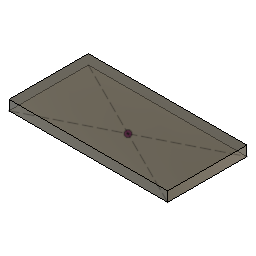
Assembly (Autodesk Fusion 360 archive; units mm, degrees)
design "PDMS Chip"
Autodesk Fusion 360 part; units mm, degrees
sketch "Sketch1" plane through (0, 0, 0) normal (0, 0, 1) x (1, 0, 0)
  line L0 (20, -10) -> (-20, -10)
  line L1 (-20, -10) -> (-20, 10)
  line L2 (-20, 10) -> (20, 10)
  line L3 (20, 10) -> (20, -10)
  line L4 (20, -10) -> (-20, 10) construction
  line L5 (-20, -10) -> (20, 10) construction
  dimension "d1" = 40
  dimension "d2" = 20
  constraint perpendicular L0 L1
  constraint parallel L0 L2
  constraint parallel L1 L3
  constraint horizontal L0
  constraint coincident L4 origin
  constraint coincident L5 origin
  measures "d1" distance of L1.end L2.end
  measures "d2" distance of L0.start L2.end
extrude "Extrude1" add sketch "Sketch1" along normal blind 2.5

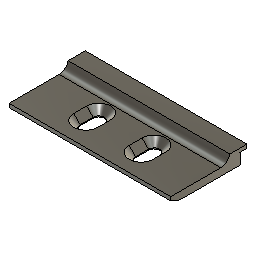
design "Microfluidic Clamp"
Autodesk Fusion 360 part; units mm, degrees
sketch "Sketch1" plane through (0, 0, 0) normal (0, 0, 1) x (1, 0, 0)
  line L0 (17.5, -7.5) -> (-17.5, -7.5)
  line L1 (-17.5, -7.5) -> (-17.5, 7.5)
  line L2 (-17.5, 7.5) -> (17.5, 7.5)
  line L3 (17.5, 7.5) -> (17.5, -7.5)
  line L4 (17.5, -7.5) -> (-17.5, 7.5) construction
  line L5 (-17.5, -7.5) -> (17.5, 7.5) construction
  dimension "d1" = 35
  dimension "d2" = 15
  constraint perpendicular L0 L1
  constraint parallel L0 L2
  constraint parallel L1 L3
  constraint horizontal L0
  constraint coincident L4 origin
  constraint coincident L5 origin
  measures "d1" distance of L1.end L2.end
  measures "d2" distance of L0.start L2.end
extrude "Extrude1" add sketch "Sketch1" along normal blind 1.6
sketch "Sketch2" plane through (17.5, 0, 0) normal (1, 0, 0) x (0, 1, 0)
  line L0 (-7.5, 0) -> (7.5, 0)
  line L1 (7.5, 0) -> (7.5, 1.6)
  line L2 (7.5, 1.6) -> (-7.5, 1.6)
  line L3 (-7.5, 1.6) -> (-7.5, 0)
  line L4 (-5.5, 0) -> (-7.5, 0.8)
  line L5 (-7.5, 0.8) -> (-7.5, 0)
  line L6 (-7.5, 0) -> (-5.5, 0)
  dimension "d5" = 2
  constraint coincident L0 L4.start
  constraint midpoint L3 L4.end
  constraint coincident L0.start L3.end
  measures "d5" distance of L4.start L0.start
extrude "Extrude2" cut sketch "Sketch2" against normal up to surface (35 mm away) contours L0 L3 L4 L5 L6
sketch "Sketch3" plane through (0, 0, 1.6) normal (0, 0, 1) x (-1, 0, 0)
  line L0 (-17.5, -7.5) -> (17.5, -7.5)
  line L1 (17.5, -7.5) -> (17.5, 7.5)
  line L2 (17.5, 7.5) -> (-17.5, 7.5)
  line L3 (-17.5, 7.5) -> (-17.5, -7.5)
  line L4 (17.5, -7.5) -> (-17.5, -7.5)
  line L5 (-17.5, -7.5) -> (-17.5, -5.3)
  line L6 (-17.5, -5.3) -> (17.5, -5.3)
  line L7 (17.5, -5.3) -> (17.5, -7.5)
  dimension "d8" = 2.2
  constraint horizontal L4
  constraint vertical L5
  constraint horizontal L6
  constraint vertical L7
  constraint coincident L3 L5.end
  constraint coincident L0.end L1.start
  measures "d8" distance of L0.start L5.end
extrude "Extrude3" add sketch "Sketch3" along normal blind 1.6 contours L0 L1 L3 L4 L5 L6 L7
fillet "Fillet1" radius 2 1 edges at (0, 5.3, 1.6)
sketch "Sketch4" plane through (0, 7.5, 0) normal (0, 1, 0) x (-1, 0, 0)
  line L0 (-17.5, 0) -> (17.5, 0)
  line L1 (17.5, 0) -> (17.5, 3.2)
  line L2 (17.5, 3.2) -> (-17.5, 3.2)
  line L3 (-17.5, 3.2) -> (-17.5, 0)
  line L4 (-17.5, 3.2) -> (17.5, 3.2)
  line L5 (17.5, 3.2) -> (17.5, 2.4)
  line L6 (17.5, 2.4) -> (-17.5, 2.4)
  line L7 (-17.5, 2.4) -> (-17.5, 3.2)
  line L8 (17.5, 1.6) -> (17.5, 3.2)
  dimension "d12" = 1
  constraint horizontal L4
  constraint vertical L5
  constraint horizontal L6
  constraint vertical L7
  constraint midpoint L5.end L8
  constraint coincident L2.end L3.start
extrude "Extrude4" add sketch "Sketch4" along normal blind 1.5 contours L1 L2 L3 L4 L5 L6 L7 L8
sketch "Sketch5" plane through (0, 0, 1.6) normal (0, 0, 1) x (-1, 0, 0)
  line L0 (-17.5, -3.3404) -> (17.5, -3.3404)
  line L1 (17.5, -3.3404) -> (17.5, 7.5)
  line L2 (17.5, 7.5) -> (-17.5, 7.5)
  line L3 (-17.5, 7.5) -> (-17.5, -3.3404)
  line L4 (6, 1) -> (-6, 1)
  line L5 (4.8, 2.4) -> (7.2, 2.4)
  line L6 (7.2, 2.4) -> (7.2, -0.4)
  line L7 (7.2, -0.4) -> (4.8, -0.4)
  line L8 (4.8, -0.4) -> (4.8, 2.4)
  line L9 (4.8, 2.4) -> (7.2, -0.4) construction
  line L10 (7.2, 2.4) -> (4.8, -0.4) construction
  arc A0 (4.8, -0.4) -> (7.2, -0.4) centre (6, -0.4) ccw
  arc A1 (7.2, 2.4) -> (4.8, 2.4) centre (6, 2.4) ccw
  line L11 (0, -1.5) -> (0, 7.5)
  arc A2 (-4.8, 2.4) -> (-7.2, 2.4) centre (-6, 2.4) ccw
  arc A3 (-7.2, -0.4) -> (-4.8, -0.4) centre (-6, -0.4) ccw
  line L12 (-4.8, 2.4) -> (-7.2, 2.4)
  line L13 (-4.8, 2.4) -> (-7.2, -0.4) construction
  line L14 (-4.8, -0.4) -> (-4.8, 2.4)
  line L15 (-7.2, 2.4) -> (-7.2, -0.4)
  line L16 (-7.2, 2.4) -> (-4.8, -0.4) construction
  line L17 (-7.2, -0.4) -> (-4.8, -0.4)
  line L18 (17.5, -7.5) -> (-17.5, -7.5)
  point P0 (0, 1)
  point P1 (6, 1)
  point P2 (-6, 1)
  point P3 (-6, 1)
  dimension "d15" = 12
  dimension "d18" = 2.4
  dimension "d19" = 2.8
  dimension "d20" = 1.2
  dimension "d21" = 1.2
  dimension "d25" = 8.5
  constraint parallel L0 L4
  constraint midpoint L4 P0
  constraint vertical origin P0
  constraint perpendicular L5 L6
  constraint parallel L5 L7
  constraint parallel L6 L8
  constraint horizontal L5
  constraint coincident L9 P1
  constraint coincident L10 P1
  constraint coincident P1 L4.start
  constraint midpoint L7 A0.centre
  constraint midpoint L5 A1.centre
  constraint midpoint L2 L11.end
  constraint perpendicular L2 L11
  constraint symmetric P1 L11 P3
  constraint symmetric L5.start L11 A2.start
  constraint symmetric L5.end L11 A2.end
  constraint symmetric L6.end L11 A3.start
  constraint symmetric L7.end L11 A3.end
  constraint symmetric A0 L11 A3
  constraint symmetric A1 L11 A2
  measures "d15" distance of P1 P3
  measures "d18" distance of L5.start L5.end
  measures "d19" distance of L5.end L6.end
  measures "d20" radius of A0
  measures "d21" radius of A1
  measures "d25" distance of L4 L18
extrude "Extrude5" cut sketch "Sketch5" against normal up to surface (1.6 mm away) contours L5 A1 | L5 L6 L7 L8 | L7 A0 | A2 L12 | L12 L14 L15 L17 | A3 L17
chamfer "Chamfer1" distance 1.4 angle 45 8 edges at (-6, -3.6, 1.6) (-7.2, -1, 1.6) (-6, 1.6, 1.6) (-4.8, -1, 1.6) (4.8, -1, 1.6) (6, 1.6, 1.6) (7.2, -1, 1.6) (6, -3.6, 1.6)
fillet "Fillet2" radius 1 1 edges at (0, -5.5, 0)

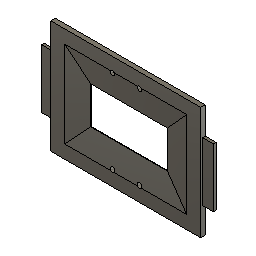
design "Microfluidic TIRF Support"
Autodesk Fusion 360 part; units mm, degrees
sketch "Sketch1" plane through (0, 0, 0) normal (0, 0, 1) x (1, 0, 0) in component "TIRF Support"
  line L0 (0, 0) -> (76, 0)
  line L1 (76, 0) -> (76, 50)
  line L2 (76, 50) -> (0, 50)
  line L3 (0, 50) -> (0, 0)
  line L4 (4.8, 38) -> (-4.8, 38)
  line L5 (-4.8, 38) -> (-4.8, 12)
  line L6 (-4.8, 12) -> (4.8, 12)
  line L7 (4.8, 12) -> (4.8, 38)
  line L8 (4.8, 38) -> (-4.8, 12) construction
  line L9 (-4.8, 38) -> (4.8, 12) construction
  line L10 (71.2, 38) -> (80.8, 38)
  line L11 (80.8, 38) -> (80.8, 12)
  line L12 (80.8, 12) -> (71.2, 12)
  line L13 (71.2, 12) -> (71.2, 38)
  line L14 (71.2, 38) -> (80.8, 12) construction
  line L15 (80.8, 38) -> (71.2, 12) construction
  line L16 (4.8, 50) -> (4.8, 0)
  line L17 (71.2, 50) -> (71.2, 0)
  line L18 (4.8, 0) -> (71.2, 50) construction
  line L19 (4.8, 50) -> (71.2, 0) construction
  point P0 (0, 25)
  point P1 (76, 25)
  point P2 (38, 25)
  dimension "d1" = 76
  dimension "d2" = 50
  dimension "d3" = 26
  dimension "d4" = 26
  dimension "d5" = 4.8
  dimension "d6" = 4.8
  constraint horizontal L0
  constraint vertical L1
  constraint horizontal L2
  constraint vertical L3
  constraint coincident L0.start L3.end
  constraint perpendicular L4 L5
  constraint parallel L4 L6
  constraint parallel L5 L7
  constraint horizontal L4
  constraint coincident L8 P0
  constraint coincident L9 P0
  constraint midpoint L3 P0
  constraint perpendicular L10 L11
  constraint parallel L10 L12
  constraint parallel L11 L13
  constraint horizontal L10
  constraint coincident L14 P1
  constraint coincident L15 P1
  constraint midpoint L1 P1
  constraint coincident L2 L16.start
  constraint coincident L0 L16.end
  constraint perpendicular L0 L16
  constraint coincident L2 L17.start
  constraint perpendicular L2 L17
  constraint coincident L0 L17.end
  constraint collinear L7 L16
  constraint collinear L13 L17
  constraint midpoint L18 P2
  measures "d1" horizontal distance of L0.start L0.end
  measures "d2" vertical distance of L0.start L2.end
  measures "d3" vertical distance of L4.end L5.end
  measures "d4" vertical distance of L10.end L11.end
  measures "d5" distance of L3 L6.end
  measures "d6" distance of L1 L11
extrude "Extrude1" add sketch "Sketch1" along normal blind 2 contours L0 L2 L7 L13 L16 L17 | L3 L4 L6 L7 L16 | L1 L10 L12 L13 L17 in component "TIRF Support"
sketch "Sketch2" plane through (0, 0, 2) normal (0, 0, 1) x (1, 0, 0) in component "TIRF Support"
  line L0 (4.8, 50) -> (4.8, 38)
  line L1 (4.8, 38) -> (0, 38)
  line L2 (0, 38) -> (0, 12)
  line L3 (0, 12) -> (4.8, 12)
  line L4 (4.8, 12) -> (4.8, 0)
  line L5 (4.8, 0) -> (71.2, 0)
  line L6 (71.2, 0) -> (71.2, 12)
  line L7 (71.2, 12) -> (76, 12)
  line L8 (76, 12) -> (76, 38)
  line L9 (76, 38) -> (71.2, 38)
  line L10 (71.2, 38) -> (71.2, 50)
  line L11 (71.2, 50) -> (4.8, 50)
  line L12 (0, 38) -> (4.8, 38)
  line L13 (4.8, 38) -> (4.8, 12)
  line L14 (4.8, 12) -> (0, 12)
  line L15 (0, 12) -> (0, 38)
  line L16 (71.2, 12) -> (76, 12)
  line L17 (76, 12) -> (76, 38)
  line L18 (76, 38) -> (71.2, 38)
  line L19 (71.2, 38) -> (71.2, 12)
  constraint horizontal L12
  constraint vertical L13
  constraint horizontal L14
  constraint vertical L15
  constraint coincident L3.end L4.start
  constraint coincident L1.end L2.start
  constraint horizontal L16
  constraint vertical L17
  constraint horizontal L18
  constraint vertical L19
  constraint coincident L8.end L9.start
  constraint coincident L6.end L7.start
extrude "Extrude2" cut sketch "Sketch2" against normal blind 0.8 contours L1 L2 L3 L12 L13 L14 L15 | L7 L8 L9 L16 L17 L18 L19 in component "TIRF Support"
sketch "Sketch3" plane through (0, 0, 0) normal (0, 0, 1) x (1, 0, 0) in component "TIRF Support"
  line L0 (71.2, 0) -> (4.8, 50)
  line L1 (4.8, 0) -> (71.2, 50)
  line L2 (17.75, 13.75) -> (58.25, 13.75)
  line L3 (58.25, 13.75) -> (58.25, 36.25)
  line L4 (58.25, 36.25) -> (17.75, 36.25)
  line L5 (17.75, 36.25) -> (17.75, 13.75)
  line L6 (17.75, 13.75) -> (58.25, 36.25) construction
  line L7 (58.25, 13.75) -> (17.75, 36.25) construction
  point P0 (71.2, 0)
  point P1 (4.8, 50)
  point P2 (4.8, 0)
  point P3 (71.2, 50)
  point P4 (38, 25)
  dimension "d11" = 22.5
  dimension "d12" = 40.5
  constraint coincident P0 L0.start
  constraint coincident P1 L0.end
  constraint coincident P2 L1.start
  constraint coincident P3 L1.end
  constraint perpendicular L2 L3
  constraint parallel L2 L4
  constraint parallel L3 L5
  constraint horizontal L2
  constraint coincident L6 P4
  constraint coincident L7 P4
  constraint midpoint L1 P4
  measures "d11" vertical distance of L2.end L3.end
  measures "d12" horizontal distance of L2.start L2.end
extrude "Extrude3" cut sketch "Sketch3" along normal blind 0.3 in component "TIRF Support"
sketch "Sketch4" plane through (0, 0, 0.3) normal (0, 0, -1) x (-1, 0, 0) in component "TIRF Support"
  line L0 (-17.75, 13.75) -> (-17.75, 36.25)
  line L1 (-17.75, 36.25) -> (-58.25, 36.25)
  line L2 (-58.25, 36.25) -> (-58.25, 13.75)
  line L3 (-58.25, 13.75) -> (-17.75, 13.75)
  line L4 (-58.25, 13.75) -> (-17.75, 36.25) construction
  line L5 (-58.25, 36.25) -> (-17.75, 13.75) construction
  line L6 (-21, 16.75) -> (-55, 16.75)
  line L7 (-55, 16.75) -> (-55, 33.25)
  line L8 (-55, 33.25) -> (-21, 33.25)
  line L9 (-21, 33.25) -> (-21, 16.75)
  line L10 (-21, 16.75) -> (-55, 33.25) construction
  line L11 (-55, 16.75) -> (-21, 33.25) construction
  point P0 (-38, 25)
  dimension "d15" = 34
  dimension "d16" = 16.5
  constraint coincident L2.end L3.start
  constraint coincident L0.end L1.start
  constraint coincident L1.end L2.start
  constraint coincident L0.start L3.end
  constraint perpendicular L6 L7
  constraint parallel L6 L8
  constraint parallel L7 L9
  constraint horizontal L6
  constraint coincident L10 P0
  constraint coincident L11 P0
  constraint midpoint L4 P0
  measures "d15" horizontal distance of L6.start L6.end
  measures "d16" vertical distance of L6.end L7.end
extrude "Extrude7" cut sketch "Sketch4" against normal blind 0.25 contours L6 L7 L8 L9 in component "TIRF Support"
sketch "Sketch5" plane through (0, 0, 2) normal (0, 0, 1) x (1, 0, 0) in component "TIRF Support"
  line L0 (4.8, 50) -> (4.8, 0)
  line L1 (4.8, 0) -> (71.2, 0)
  line L2 (71.2, 0) -> (71.2, 50)
  line L3 (71.2, 50) -> (4.8, 50)
  line L4 (65, 44.141) -> (11, 44.141)
  line L5 (11, 44.141) -> (11, 5.859)
  line L6 (11, 5.859) -> (65, 5.859)
  line L7 (65, 5.859) -> (65, 44.141)
  line L8 (65, 44.141) -> (11, 5.859) construction
  line L9 (11, 44.141) -> (65, 5.859) construction
  line L10 (21, 33.25) -> (21, 16.75)
  point P0 (38, 25)
  point P1 (38, 25)
  dimension "d18" = 38.282
  dimension "d74" = 10
  constraint perpendicular L4 L5
  constraint parallel L4 L6
  constraint parallel L5 L7
  constraint horizontal L4
  constraint coincident L8 P1
  constraint coincident L9 P1
  constraint coincident P1 P0
  measures "d18" vertical distance of L4.end L5.end
  measures "d74" distance of L5 L10
sketch "Sketch2 (2)" plane through (0, 0, 0) normal (0, 0, -1) x (-1, 0, 0)
  line L0 (-58.25, 36.25) -> (-17.75, 36.25)
  line L1 (-17.75, 36.25) -> (-17.75, 13.75)
  line L2 (-17.75, 13.75) -> (-58.25, 13.75)
  line L3 (-58.25, 13.75) -> (-58.25, 36.25)
  line L4 (-4.8, 38) -> (-4.8, 50)
  line L5 (-4.8, 50) -> (-71.2, 50)
  line L6 (-71.2, 50) -> (-71.2, 38)
  line L7 (-71.2, 38) -> (-76, 38)
  line L8 (-76, 38) -> (-76, 12)
  line L9 (-76, 12) -> (-71.2, 12)
  line L10 (-71.2, 12) -> (-71.2, 0)
  line L11 (-71.2, 0) -> (-4.8, 0)
  line L12 (-4.8, 0) -> (-4.8, 12)
  line L13 (-4.8, 12) -> (0, 12)
  line L14 (0, 12) -> (0, 38)
  line L15 (0, 38) -> (-4.8, 38)
  line L16 (-58.25, 40.25) -> (-54.25, 40.25)
  line L17 (-54.25, 40.25) -> (-54.25, 9.75)
  line L18 (-54.25, 9.75) -> (-58.25, 9.75)
  line L19 (-58.25, 9.75) -> (-58.25, 40.25)
  line L20 (-17.75, 40.25) -> (-21.75, 40.25)
  line L21 (-21.75, 40.25) -> (-21.75, 9.75)
  line L22 (-21.75, 9.75) -> (-17.75, 9.75)
  line L23 (-17.75, 9.75) -> (-17.75, 40.25)
  dimension "d38" = 4
  dimension "d39" = 4
  dimension "d40" = 4
  dimension "d41" = 4
  dimension "d42" = 4
  dimension "d43" = 4
  constraint perpendicular L16 L17
  constraint parallel L16 L18
  constraint parallel L17 L19
  constraint perpendicular L20 L21
  constraint parallel L20 L22
  constraint parallel L21 L23
  constraint collinear L3 L19
  constraint collinear L1 L23
  measures "d38" horizontal distance of L16.start L16.end
  measures "d39" horizontal distance of L20.start L20.end
  measures "d40" distance of L2 L18
  measures "d41" distance of L0 L16
  measures "d42" distance of L0 L20
  measures "d43" distance of L2 L22
loft "Loft2" cut profiles "Sketch5" section 1 contours L4 L5 L6 L7 section 2 face at (32.3333, 22.25, 0.55) in component "TIRF Support"
sketch "Sketch3 (2)" plane through (-13.1789, -7.5617, 0) normal (0, 0, -1) x (-1, 0, 0)
  line L0 (-71.4289, 43.8117) -> (-30.9289, 43.8117)
  line L1 (-30.9289, 43.8117) -> (-30.9289, 21.3117)
  line L2 (-30.9289, 21.3117) -> (-71.4289, 21.3117)
  line L3 (-71.4289, 21.3117) -> (-71.4289, 43.8117)
  line L4 (-17.9789, 45.5617) -> (-17.9789, 57.5617)
  line L5 (-17.9789, 57.5617) -> (-84.3789, 57.5617)
  line L6 (-84.3789, 57.5617) -> (-84.3789, 45.5617)
  line L7 (-84.3789, 45.5617) -> (-89.1789, 45.5617)
  line L8 (-89.1789, 45.5617) -> (-89.1789, 19.5617)
  line L9 (-89.1789, 19.5617) -> (-84.3789, 19.5617)
  line L10 (-84.3789, 19.5617) -> (-84.3789, 7.5617)
  line L11 (-84.3789, 7.5617) -> (-17.9789, 7.5617)
  line L12 (-17.9789, 7.5617) -> (-17.9789, 19.5617)
  line L13 (-17.9789, 19.5617) -> (-13.1789, 19.5617)
  line L14 (-13.1789, 19.5617) -> (-13.1789, 45.5617)
  line L15 (-13.1789, 45.5617) -> (-17.9789, 45.5617)
  line L16 (-68.1789, 24.3117) -> (-68.1789, 40.8117)
  line L17 (-68.1789, 40.8117) -> (-34.1789, 40.8117)
  line L18 (-34.1789, 40.8117) -> (-34.1789, 24.3117)
  line L19 (-34.1789, 24.3117) -> (-68.1789, 24.3117)
  line L20 (-30.9289, 21.3117) -> (-30.9289, 43.8117)
  line L21 (-30.9289, 43.8117) -> (-71.4289, 43.8117)
  line L22 (-71.4289, 43.8117) -> (-71.4289, 21.3117)
  line L23 (-71.4289, 21.3117) -> (-30.9289, 21.3117)
  line L24 (-68.1789, 24.3117) -> (-34.1789, 40.8117) construction
  line L25 (-68.1789, 40.8117) -> (-34.1789, 24.3117) construction
  line L26 (-45.1789, 51.0617) -> (-57.1789, 51.0617) construction
  line L27 (-57.1789, 51.0617) -> (-57.1789, 14.0617) construction
  line L28 (-57.1789, 14.0617) -> (-45.1789, 14.0617) construction
  line L29 (-45.1789, 14.0617) -> (-45.1789, 51.0617) construction
  line L30 (-45.1789, 51.0617) -> (-57.1789, 14.0617) construction
  line L31 (-57.1789, 51.0617) -> (-45.1789, 14.0617) construction
  circle A0 centre (-57.1789, 51.0617) radius 1.025
  circle A1 centre (-45.1789, 51.0617) radius 1.025
  circle A2 centre (-45.1789, 14.0617) radius 1.025
  circle A3 centre (-57.1789, 14.0617) radius 1.025
  point P0 (-51.1789, 32.5617)
  dimension "d55" = 12
  dimension "d56" = 37
  dimension "d57" = 2.05
  dimension "d58" = 2.05
  dimension "d59" = 2.05
  dimension "d60" = 2.05
  constraint coincident L16.start L19.end
  constraint coincident L17.end L18.start
  constraint coincident L16.end L17.start
  constraint coincident L18.end L19.start
  constraint perpendicular L26 L27
  constraint parallel L26 L28
  constraint parallel L27 L29
  constraint horizontal L26
  constraint coincident L30 P0
  constraint coincident L31 P0
  constraint midpoint L25 P0
  constraint coincident L26.end L27.start
  constraint coincident L26.start L29.end
  constraint coincident L28.end L29.start
  constraint coincident L27.end L28.start
  measures "d55" horizontal distance of L26.start L26.end
  measures "d56" vertical distance of L26.end L27.end
  measures "d57" diameter of A0
  measures "d58" diameter of A1
  measures "d59" diameter of A3
  measures "d60" diameter of A2
extrude "Extrude8" cut sketch "Sketch3 (2)" against normal blind 8 contours A0 | A1 | A2 | A3 in component "TIRF Support"
sketch "Sketch4 (2)" plane through (0, 0, 0) normal (0, 0, -1) x (-1, 0, 0)
  circle A0 centre (-32, 43.5) radius 1.025
  circle A1 centre (-44, 6.5) radius 1.025
  circle A2 centre (-44, 43.5) radius 1.025
  circle A3 centre (-32, 6.5) radius 1.025
  line L0 (-58.25, 36.25) -> (-17.75, 36.25)
  line L1 (-17.75, 36.25) -> (-17.75, 13.75)
  line L2 (-17.75, 13.75) -> (-58.25, 13.75)
  line L3 (-58.25, 13.75) -> (-58.25, 36.25)
  line L4 (-4.8, 38) -> (-4.8, 50)
  line L5 (-4.8, 50) -> (-71.2, 50)
  line L6 (-71.2, 50) -> (-71.2, 38)
  line L7 (-71.2, 38) -> (-76, 38)
  line L8 (-76, 38) -> (-76, 12)
  line L9 (-76, 12) -> (-71.2, 12)
  line L10 (-71.2, 12) -> (-71.2, 0)
  line L11 (-71.2, 0) -> (-4.8, 0)
  line L12 (-4.8, 0) -> (-4.8, 12)
  line L13 (-4.8, 12) -> (0, 12)
  line L14 (0, 12) -> (0, 38)
  line L15 (0, 38) -> (-4.8, 38)
  line L16 (-60.25, 38) -> (-58.25, 38)
  line L17 (-58.25, 38) -> (-58.25, 12)
  line L18 (-58.25, 12) -> (-60.25, 12)
  line L19 (-60.25, 12) -> (-60.25, 38)
  line L20 (-17.75, 38) -> (-15.75, 38)
  line L21 (-15.75, 38) -> (-15.75, 12)
  line L22 (-15.75, 12) -> (-17.75, 12)
  line L23 (-17.75, 12) -> (-17.75, 38)
  line L24 (-60.25, 38) -> (-58.25, 12) construction
  line L25 (-60.25, 12) -> (-58.25, 38) construction
  line L26 (-17.75, 38) -> (-15.75, 12) construction
  line L27 (-17.75, 12) -> (-15.75, 38) construction
  line L28 (-76, 25) -> (0, 25) construction
  point P0 (-59.25, 25)
  point P1 (-16.75, 25)
  dimension "d63" = 2
  dimension "d64" = 2
  dimension "d67" = 26
  dimension "d68" = 26
  constraint horizontal L16
  constraint vertical L17
  constraint horizontal L18
  constraint vertical L19
  constraint horizontal L20
  constraint vertical L21
  constraint horizontal L22
  constraint vertical L23
  constraint midpoint L8 L28.start
  constraint midpoint L14 L28.end
  constraint midpoint L25 P0
  constraint midpoint L27 P1
  constraint coincident L28 P1
  constraint coincident L28 P0
  constraint collinear L3 L17
  constraint collinear L1 L23
  measures "d63" horizontal distance of L17.end L18.end
  measures "d64" horizontal distance of L21.end L22.end
  measures "d67" vertical distance of L16.start L18.end
  measures "d68" vertical distance of L20.end L21.end
extrude "Extrude9" [suppressed] in component "TIRF Support"
fillet "Fillet6" [suppressed] in component "TIRF Support"
ref_plane "WorkPlane1" through (38, 25, 1) normal (0, -1, 0) x (1, 0, 0)
component "TIRF Support" placed x (1, 0, 0) y (0, 1, 0) z (0, 0, 1) at (0, 0, 0)
equation "d4 = d3"
equation "d6 = d5"
equation "d39 = d38"
equation "d40 = d41"
equation "d41 = d38"
equation "d42 = d41"
equation "d43 = d41"
equation "d64 = d63"
